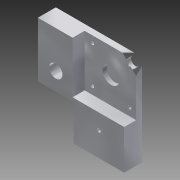
# Autodesk Inventor part: wooden1
Saved by Autodesk Inventor 2015 (Build 190159000, 159)
## iProperties
Created: 2016-04-26
Part Number: wooden1
Material: Aluminum 6061
Document SubType Name: Modeling
Designer: Kostya
Density: 2.7 g/cm^3
Appearance: Aluminum - Flat
Author: Kostya
Autodesk Inventor part; units mm, degrees
ref_plane "YZ Plane" through (0, 0, 0) normal (1, 0, 0) x (0, 1, 0)
ref_plane "XZ Plane" through (0, 0, 0) normal (0, 1, 0) x (-1, 0, 0)
ref_plane "XY Plane" through (0, 0, 0) normal (0, 0, 1) x (1, 0, 0)
sketch "Sketch1" plane through (0, 0, 0) normal (0, 1, 0) x (-1, 0, 0)
  line L0 (-12, 16) -> (60, 16)
  line L1 (60, 16) -> (60, -30)
  line L2 (60, -30) -> (30, -30)
  line L3 (30, -30) -> (30, -60)
  line L4 (30, -60) -> (-12, -60)
  line L5 (-12, -60) -> (-12, 16)
  dimension "d0" = 72
  dimension "d1" = 46
  dimension "d2" = 30
  dimension "d3" = 30
  dimension "d4" = 42
  constraints: 12 end point, 4 perpendicular
  measures "d0" distance of L0.start L0.end
  measures "d1" distance of L0.end L1.end
  measures "d2" distance of L1.end L2.end
  measures "d3" distance of L2.end L3.end
  measures "d4" distance of L3.end L4.end
extrude "Extrusion1" add sketch "Sketch1" along normal blind 15
sketch "Sketch13" plane through (0, 15, 0) normal (0, 1, 0) x (1, 0, 0)
  circle A0 centre (6.5, -10.5) radius 3.75
  circle A1 centre (-24.5, -10.5) radius 3.75
  circle A2 centre (6.5, 20.5) radius 3.75
  circle A3 centre (-24.5, 20.5) radius 3.75
  line L0 (-60, -16) -> (12, -16) projected
  point P0 (0, 0)
  dimension "d57" = 7.5
  dimension "d58" = 7.5
  dimension "d59" = 7.5
  dimension "d60" = 7.5
  dimension "d68" = 5.5
  dimension "d69" = 31
  constraints: 4 centre point, 2 horizontal alignment, 2 vertical alignment
  measures "d57" diameter of A0
  measures "d58" diameter of A1
  measures "d59" diameter of A2
  measures "d60" diameter of A3
  measures "d68" distance from line of L0 A0.centre
  measures "d69" distance of A2.centre A0.centre
extrude "Extrusion7" cut sketch "Sketch13" against normal blind 4
sketch "Sketch14" plane through (6.5, 11, 10.5) normal (0, 1, 0) x (1, 0, 0)
  circle A0 centre (0, 0) radius 1.5
  circle A1 centre (-31, 0) radius 1.5
  circle A2 centre (0, 31) radius 3.75 projected
  circle A3 centre (0, 31) radius 1.5
  circle A4 centre (-31, 31) radius 1.5
  point P0 (-6.5, 10.5)
  dimension "d63" = 3
  dimension "d64" = 3
  dimension "d65" = 3
  constraints: 4 centre point, 1 coincident
  measures "d63" diameter of A0
  measures "d64" diameter of A1
  measures "d65" diameter of A3
extrude "Extrusion8" cut sketch "Sketch14" against normal up to next contours A0 | A1 | A3 | A4
sketch "Sketch15" plane through (0, 0, 0) normal (0, -1, 0) x (1, 0, 0)
  circle A0 centre (-45, -15) radius 3
  circle A1 centre (-9, -40) radius 1.5
  line L0 (-30, -60) -> (12, -60) projected
  point P0 (0, 0)
  dimension "d72" = 6
  dimension "d73" = 3
  dimension "d89" = 20
  constraints: 2 centre point
  measures "d72" diameter of A0
  measures "d73" diameter of A1
  measures "d89" distance from line of L0 A1.centre
extrude "Extrusion10" cut sketch "Sketch15" against normal up to next
sketch "Sketch16" plane through (0, 0, 0) normal (0, -1, 0) x (1, 0, 0)
  circle A0 centre (-9, -5) radius 7
  point P0 (0, 0)
  dimension "d79" = 14
  constraints: 1 centre point
  measures "d79" diameter of A0
extrude "Extrusion11" cut sketch "Sketch16" against normal blind 4
sketch "Sketch17" plane through (0, 0, 0) normal (0, -1, 0) x (1, 0, 0)
  line L0 (12, 16) -> (-31, 16)
  line L1 (-31, 16) -> (-31, -27)
  line L2 (-31, -27) -> (12, -27)
  line L3 (12, -27) -> (12, 16)
  point P0 (0, 0)
  dimension "d82" = 43
  dimension "d83" = 43
  constraints: 8 end point, 2 parallel, 1 horizontal, 1 perpendicular
  measures "d82" distance of L2.end L1.end
  measures "d83" distance of L1.end L0.end
extrude "Extrusion12" cut sketch "Sketch17" against normal blind 10
sketch "Sketch18" plane through (0, 10, 0) normal (0, -1, 0) x (1, 0, 0)
  circle A0 centre (-9, -5) radius 7
  point P0 (0, 0)
  dimension "d86" = 14
  constraints: 1 centre point
  measures "d86" diameter of A0
extrude "Extrusion13" cut sketch "Sketch18" against normal blind 3.5
sketch "Sketch19" plane through (0, 0, 0) normal (0, -1, 0) x (1, 0, 0)
  circle A0 centre (-45, -15) radius 5.5
  point P0 (0, 0)
  dimension "d90" = 11
  constraints: 1 centre point
  measures "d90" diameter of A0
extrude "Extrusion14" cut sketch "Sketch19" against normal blind 11
sketch "Sketch3" plane through (0, 15, 0) normal (0, 1, 0) x (1, 0, 0)
  point P0 (-45, 15)
body "Solid1"
